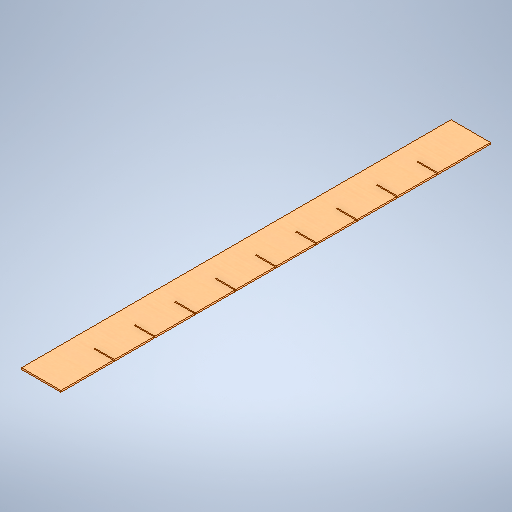
# Autodesk Inventor part: Base
Saved by Autodesk Inventor 2025.2 (Build 292293000, 293)
## iProperties
Created: 2025-05-12
Part Number: Base
Material: Wood (Cherry)
Document SubType Name: Modeling
Designer: USER
Density: 0.63 g/cm^3
Appearance: Cherry - Natural Low Gloss
Author: USER
Autodesk Inventor part; units mm, degrees
ref_plane "YZ Plane" through (0, 0, 0) normal (1, 0, 0) x (0, 1, 0)
ref_plane "XZ Plane" through (0, 0, 0) normal (0, 1, 0) x (-1, 0, 0)
ref_plane "XY Plane" through (0, 0, 0) normal (0, 0, 1) x (1, 0, 0)
sketch "Sketch1" plane through (0, 0, 0) normal (0, 1, 0) x (-1, 0, 0)
  line L0 (0, 0) -> (150, 0)
  line L1 (150, 0) -> (150, -1636)
  line L2 (150, -1636) -> (0, -1636)
  line L3 (0, -1636) -> (0, 0)
  dimension "d0" = 150
  dimension "d1" = 1636
  constraints: 8 end point, 2 parallel, 1 horizontal, 1 perpendicular
  measures "d0" distance of L1.end L2.end
  measures "d1" distance of L0.end L1.end
extrude "Extrusion1" add sketch "Sketch1" along normal blind 6
sketch "Sketch2" plane through (0, 6, 0) normal (0, 1, 0) x (1, 0, 0)
  line L0 (-150, 200) -> (0, 200)
  line L1 (-150, 0) -> (0, 0) projected
  line L2 (-150, 204) -> (0, 204)
  line L3 (-75, 200) -> (-75, 204)
  line L4 (-150, 354) -> (0, 354)
  line L5 (-150, 358) -> (0, 358)
  line L6 (-75, 354) -> (-75, 358)
  line L7 (-150, 508) -> (0, 508)
  line L8 (-150, 512) -> (0, 512)
  line L9 (-75, 508) -> (-75, 512)
  line L10 (-150, 662) -> (0, 662)
  line L11 (-150, 666) -> (0, 666)
  line L12 (-75, 662) -> (-75, 666)
  line L13 (-150, 816) -> (0, 816)
  line L14 (-150, 820) -> (0, 820)
  line L15 (-75, 816) -> (-75, 820)
  line L16 (-150, 970) -> (0, 970)
  line L17 (-150, 974) -> (0, 974)
  line L18 (-75, 970) -> (-75, 974)
  line L19 (-150, 1436) -> (0, 1436)
  line L20 (-150, 1432) -> (0, 1432)
  line L21 (-150, 1282) -> (0, 1282)
  line L22 (-150, 1278) -> (0, 1278)
  line L23 (-150, 1128) -> (0, 1128)
  line L24 (-150, 1124) -> (0, 1124)
  line L25 (-75, 1124) -> (-75, 1128)
  line L26 (-75, 1278) -> (-75, 1282)
  line L27 (-75, 1432) -> (-75, 1436)
  line L28 (0, 0) -> (0, 1636) projected
  line L29 (0, 0) -> (0, 1636)
  dimension "d4" = 200
  dimension "d5" = 4
  dimension "d6" = 150
  dimension "d7" = 4
  dimension "d8" = 150
  dimension "d9" = 4
  dimension "d10" = 150
  dimension "d11" = 4
  dimension "d12" = 150
  dimension "d13" = 4
  dimension "d14" = 150
  dimension "d15" = 4
  dimension "d19" = 150
  dimension "d21" = 150
  dimension "d22" = 150
  dimension "d40" = 4
  dimension "d41" = 4
  dimension "d42" = 4
  constraints: 56 end point, 18 midpoint, 3 horizontal, 2 vertical, 1 other
  measures "d4" distance between parallel lines of L0 L1
  measures "d5" distance between parallel lines of L0 L2
  measures "d6" distance between parallel lines of L4 L2
  measures "d7" distance between parallel lines of L4 L5
  measures "d8" distance between parallel lines of L7 L5
  measures "d9" distance from line of L9.end L7
  measures "d10" distance between parallel lines of L10 L8
  measures "d11" distance between parallel lines of L10 L11
  measures "d12" distance between parallel lines of L11 L13
  measures "d13" distance between parallel lines of L13 L14
  measures "d14" distance between parallel lines of L14 L16
  measures "d15" distance between parallel lines of L16 L17
  measures "d19" distance between parallel lines of L17 L24
  measures "d21" distance between parallel lines of L22 L23
  measures "d22" distance between parallel lines of L20 L21
  measures "d40" distance between parallel lines of L24 L23
  measures "d41" distance between parallel lines of L21 L22
  measures "d42" distance between parallel lines of L20 L19
extrude "Extrusion2" cut sketch "Sketch2" against normal blind 6
body "Solid1"
